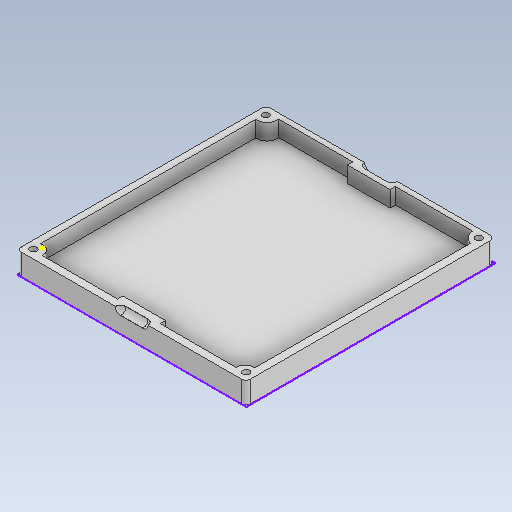
# Autodesk Inventor part: Case 1 Cover
Saved by Autodesk Inventor 2020.2 (Build 242310000, 310)
## iProperties
Created: 2019-11-25
Part Number: Case 1 Cover
Material: Generic
Document SubType Name: Modeling
Designer: athiy
Density: 1 g/cm^3
Appearance: Default
Author: athiy
Autodesk Inventor part; units mm, degrees
ref_plane "YZ Plane" through (0, 0, 0) normal (1, 0, 0) x (0, 1, 0)
ref_plane "XZ Plane" through (0, 0, 0) normal (0, 1, 0) x (-1, 0, 0)
ref_plane "XY Plane" through (0, 0, 0) normal (0, 0, 1) x (1, 0, 0)
sketch "Sketch1" plane through (0, 0, 0) normal (0, 1, 0) x (-1, 0, 0)
  line L0 (-81.2549, 4.894) -> (-81.2549, -88.547)
  line L1 (4.6415, -88.547) -> (4.6415, 4.894)
  line L2 (4.6415, -88.547) -> (-81.2549, -88.547)
  line L3 (4.6415, 4.894) -> (-81.2549, 4.894)
  point P0 (0, 0)
  constraints: 8 end point, 1 horizontal, 1 perpendicular, 1 vertical
extrude "Extrusion1" add sketch "Sketch1" along normal blind 8
fillet "Fillet1" radius 2 1 edges at (81.2549, 4, -88.547)
sketch "Sketch2" plane through (0, 8, 0) normal (0, 1, 0) x (1, 0, 0)
  point P0 (0, 0)
extrude "Extrusion2" [suppressed]
fillet "Fillet2" [suppressed]
sketch "Sketch3" plane through (0, 2.25, 0) normal (0, 1, 0) x (1, 0, 0)
  point P0 (0, 0)
sketch "Sketch4" plane through (0, 2.25, 0) normal (0, 1, 0) x (1, 0, 0)
  arc A0 (6.27, 28.88) -> (5, 27.61) centre (6.27, 27.61) ccw projected
  line L0 (6.27, 28.88) -> (30.5, 28.88)
  line L1 (6.27, 28.88) -> (30.5, 28.88) construction
  point P0 (0, 0)
  constraints: 4 end point, 1 collinear, 1 horizontal
extrude "Extrusion3" [suppressed]
sketch "Sketch5" plane through (7.5401, 2.25, -26.3758) normal (0, 1, 0) x (1, 0, 0)
  circle A0 centre (0, 0) radius 1.27
  point P0 (-7.5401, -26.3758)
  constraints: 1 centre point
extrude "Extrusion4" [suppressed]
sketch "Sketch6" plane through (7.5401, 2.25, -8.5042) normal (0, 1, 0) x (1, 0, 0)
  circle A0 centre (0, 0) radius 1.9 projected
  circle A1 centre (0, 0) radius 1.27
  point P0 (-7.5401, -8.5042)
  constraints: 1 centre point, 1 coincident
extrude "Extrusion5" [suppressed]
sketch "Sketch7" plane through (53.4599, 2.25, -26.3758) normal (0, 1, 0) x (1, 0, 0)
  circle A0 centre (0, 0) radius 1.27 projected
  circle A1 centre (0, 0) radius 1.27
  point P0 (-53.4599, -26.3758)
  constraints: 1 centre point, 1 coincident
extrude "Extrusion6" [suppressed]
sketch "Sketch8" plane through (53.4599, 2.25, -8.5042) normal (0, 1, 0) x (1, 0, 0)
  circle A0 centre (0, 0) radius 1.27 projected
  circle A1 centre (0, 0) radius 1.27
  point P0 (-53.4599, -8.5042)
  constraints: 1 centre point, 1 coincident
sketch "Sketch9" plane through (0, 8, 0) normal (0, 1, 0) x (1, 0, 0)
  line L0 (81.2549, -4.894) -> (81.2549, 86.547) projected
  point P0 (0, 0)
  point P1 (81.2549, 2)
extrude "Extrusion7" [suppressed]
fillet "Fillet3" [suppressed]
sketch "Sketch10" plane through (0, 2.25, 0) normal (0, 1, 0) x (1, 0, 0)
  line L0 (52.17, 47.7819) -> (7.87, 47.7819) projected
  line L1 (6.27, 49.3819) -> (6.27, 76.6519) projected
  line L2 (6.27, 63.0169) -> (53.77, 63.0169)
  line L3 (53.77, 76.6519) -> (53.77, 49.3819) projected
  line L4 (30.02, 47.7819) -> (30.02, 78.2519)
  line L5 (7.87, 78.2519) -> (52.17, 78.2519) projected
  point P0 (0, 0)
  constraints: 4 end point, 4 midpoint
extrude "Extrusion8" [suppressed]
extrude "Extrusion9" [suppressed]
sketch "Sketch11" plane through (9.47, 2.25, -50.9819) normal (0, 1, 0) x (1, 0, 0)
  circle A0 centre (0, 0) radius 1.6
  point P0 (-9.47, -50.9819)
  constraints: 1 centre point
extrude "Extrusion10" [suppressed]
sketch "Sketch12" plane through (9.47, 2.25, -75.0519) normal (0, 1, 0) x (1, 0, 0)
  circle A0 centre (0, 0) radius 1.6
  point P0 (-9.47, -75.0519)
  constraints: 1 centre point
extrude "Extrusion11" [suppressed]
sketch "Sketch13" plane through (50.57, 2.25, -50.9819) normal (0, 1, 0) x (1, 0, 0)
  circle A0 centre (0, 0) radius 1.6
  point P0 (-50.57, -50.9819)
  constraints: 1 centre point
extrude "Extrusion12" [suppressed]
sketch "Sketch14" plane through (50.57, 2.25, -75.0519) normal (0, 1, 0) x (1, 0, 0)
  point P0 (-50.57, -75.0519)
  point P1 (0, 0)
extrude "Extrusion13" [suppressed]
sketch "Sketch15" plane through (0, 8, 0) normal (0, 1, 0) x (1, 0, 0)
  point P0 (0, 0)
sketch "Sketch16" plane through (0, 8, 0) normal (0, 1, 0) x (1, 0, 0)
  line L0 (53.77, 74.7519) -> (71.77, 74.7519) projected
  line L1 (53.77, 74.7519) -> (71.77, 74.7519)
  line L2 (71.77, 74.7519) -> (71.77, 59.4972) projected
  line L3 (71.77, 74.7519) -> (71.77, 59.4972)
  line L4 (71.77, 59.4972) -> (53.77, 59.4972) projected
  line L5 (71.77, 59.4972) -> (53.77, 59.4972)
  circle A0 centre (-0.8495, 85.0914) radius 1.27
  line L6 (-4.6415, 88.547) -> (-4.6415, -4.894) projected
  line L7 (-4.6415, 41.8265) -> (81.2549, 41.8265)
  line L8 (81.2549, -4.894) -> (81.2549, 86.547) projected
  circle A1 centre (-0.8495, -1.4384) radius 1.27
  line L9 (-2.1195, 82.1131) -> (-2.1195, 1.3369)
  line L10 (2.1021, 86.547) -> (74.7894, 86.547)
  arc A2 (-2.1195, 82.1131) -> (2.1021, 86.547) centre (-1.6738, 85.9154) ccw
  line L11 (2.1021, -2.1183) -> (74.7894, -2.1183)
  line L12 (78.4154, 82.1131) -> (78.4154, 1.3369)
  arc A3 (74.7894, 86.547) -> (78.4154, 82.1131) centre (80.0457, 87.1459) ccw
  arc A4 (78.4154, 1.3369) -> (74.7894, -2.1183) centre (78.0984, -1.9607) ccw
  arc A5 (2.1021, -2.1183) -> (-2.1195, 1.3369) centre (-1.3126, -1.9838) ccw
  circle A6 centre (78.0984, -1.9607) radius 1.27
  circle A7 centre (78.0984, 85.6137) radius 1.27
  point P0 (0, 0)
  point P1 (79.2549, 88.547)
  constraints: 16 end point, 8 centre point, 8 point on circle, 3 collinear, 3 horizontal, 2 symmetric about line, 1 coincident, 1 midpoint, 1 parallel, 1 point on line, 1 vertical, 2 other
extrude "Extrusion14" cut sketch "Sketch16" against normal blind 6 contours L9 A2 L10 A3 L12 L7 | L7 L12 A4 L11 A5 L9
sketch "Sketch17" plane through (0, 8, 0) normal (0, 1, 0) x (1, 0, 0)
  circle A0 centre (-1.6277, -1.7597) radius 1.27
  line L0 (-4.6415, 88.547) -> (-4.6415, -4.894) projected
  line L1 (-4.6415, 41.8265) -> (80.9593, 41.8265)
  circle A1 centre (-1.6277, 85.4127) radius 1.27
  circle A2 centre (78.2293, -1.7597) radius 1.27
  circle A3 centre (78.2293, 85.4127) radius 1.27
  point P0 (0, 0)
  constraints: 4 centre point, 2 end point, 2 symmetric about line, 1 horizontal, 1 midpoint, 2 other
extrude "Extrusion15" cut sketch "Sketch17" against normal through all
fillet "Fillet4" radius 1.6 3 edges at (81.2549, 4, 4.894) (-4.6415, 4, -88.547) (-4.6415, 4, 4.894)
sketch "Sketch18" plane through (74.7894, 8, 2.1183) normal (0, 0, -1) x (-1, 0, 0)
  line L0 (-6.4655, 0) -> (-4.4655, 0) projected
  line L1 (79.4309, -8) -> (79.4309, 0) projected
  line L2 (36.4825, 0) -> (44.4825, 0)
  line L3 (44.4825, -8) -> (28.4825, -8)
  line L4 (-4.4655, -8) -> (77.8309, -8) projected
  line L5 (28.4825, -8) -> (28.4825, 0)
  line L6 (44.4825, 0) -> (38.4825, 0)
  line L7 (-4.4655, 0) -> (77.8309, 0) projected
  line L8 (44.4825, 0) -> (44.4825, -6)
  line L9 (44.4825, -6) -> (28.4825, -6)
  line L10 (72.6873, -6) -> (0, -6) projected
  line L11 (28.4825, -6) -> (28.4825, 0)
  point P0 (74.7894, -8)
  point P1 (28.4825, -6)
  dimension "d81" = 42.948
  dimension "d82" = 8
  dimension "d85" = 6
  dimension "d86" = 16
  constraints: 14 end point, 3 point on line, 1 perpendicular, 1 vertical
  measures "d81" distance of L0.start L2.start
  measures "d82" distance of L2.start L2.end
  measures "d85" distance of L2.end L8.end
  measures "d86" distance of L8.end L9.end
extrude "Extrusion16" add sketch "Sketch18" along normal blind 2
sketch "Sketch19" plane through (0, 8, 0) normal (0, 1, 0) x (1, 0, 0)
  point P0 (0, 0)
sketch "Sketch20" plane through (2.1021, 8, -86.547) normal (0, 0, 1) x (1, 0, 0)
  line L0 (-6.7435, -8) -> (-6.7435, 0) projected
  line L1 (-6.7435, 0) -> (35.7545, 0)
  line L2 (-5.1435, 0) -> (77.5529, 0) projected
  line L3 (35.7545, 0) -> (43.7545, 0)
  line L4 (28.2049, 0) -> (35.7545, 0)
  line L5 (43.7545, 0) -> (43.7545, -6)
  line L6 (0, -6) -> (72.6873, -6) projected
  line L7 (43.7545, -6) -> (27.7545, -6)
  line L8 (27.7545, -6) -> (27.7545, 0)
  point P0 (-2.1021, -8)
  dimension "d89" = 42.498
  dimension "d90" = 8
  dimension "d94" = 16
  constraints: 12 end point, 5 point on line, 1 collinear, 1 perpendicular, 1 vertical
  measures "d89" distance of L0.end L1.end
  measures "d90" distance of L1.end L3.end
  measures "d94" distance of L5.end L7.end
extrude "Extrusion17" add sketch "Sketch20" along normal blind 2
sketch "Sketch21" plane through (0, 8, 0) normal (0, 1, 0) x (1, 0, 0)
  arc A0 (42.5594, 86.5345) -> (44.5594, 88.5345) centre (42.5594, 88.5345) ccw
  line L0 (34.2677, 86.5345) -> (42.5594, 86.5345)
  line L1 (30.2832, -4.894) -> (32.2832, -4.894) construction
  arc A1 (32.2832, 88.5498) -> (34.2677, 86.5345) centre (34.2831, 88.5344) ccw
  arc A2 (34.2831, -2.894) -> (32.2832, -4.894) centre (34.2832, -4.894) ccw
  arc A3 (44.5594, -4.894) -> (42.5594, -2.894) centre (42.5594, -4.894) ccw
  line L2 (34.2831, -2.894) -> (42.5594, -2.894)
  line L3 (32.2832, -4.894) -> (44.5594, -4.894)
  point P0 (0, 0)
  dimension "d113" = 2
  dimension "d114" = 2
  constraints: 8 end point, 8 point on circle, 4 centre point, 3 horizontal
  measures "d113" radius of A2
  measures "d114" radius of A3
extrude "Extrusion18" cut sketch "Sketch21" against normal blind 2
sketch "Sketch22" plane through (0, 8, 0) normal (0, 1, 0) x (1, 0, 0)
  arc A0 (44.5594, -4.894) -> (42.5594, -2.894) centre (42.5594, -4.894) ccw projected
  line L0 (79.2549, 88.547) -> (-3.0415, 88.547) projected
  line L1 (44.5594, -4.894) -> (138.0005, -4.894) construction
  arc A1 (42.5594, 86.547) -> (44.5594, 88.547) centre (42.5594, 88.547) ccw
  arc A2 (32.3481, 88.547) -> (34.3481, 86.547) centre (34.3481, 88.547) ccw
  line L2 (42.5594, 86.547) -> (34.3481, 86.547)
  point P0 (0, 0)
  dimension "d120" = 2
  dimension "d121" = 2
  constraints: 4 end point, 4 point on circle, 2 centre point, 2 horizontal, 2 point on line
  measures "d120" radius of A1
  measures "d121" radius of A2
extrude "Extrusion19" cut sketch "Sketch22" against normal blind 2
fillet "Fillet5" radius 2 3 edges at (32.9339, 6, -87.1328) (43.9736, 6, -87.1328) (38.4538, 6, -86.547)
fillet "Fillet6" radius 1.9 3 edges at (43.9736, 6, 3.4798) (32.8689, 6, 3.4798) (38.4213, 6, 2.894)
body "Solid1"
